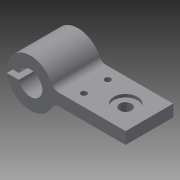
# Autodesk Inventor part: HW 5 Part 4
Saved by Autodesk Inventor 2015 (Build 190159000, 159)
## iProperties
Created: 2016-02-07
Part Number: HW 5 Part 4
Material: Generic
Document SubType Name: Modeling
Designer: Melissa
Density: 1 g/cm^3
Appearance: Default
Author: Melissa
Autodesk Inventor part; units mm, degrees
ref_plane "YZ Plane" through (0, 0, 0) normal (1, 0, 0) x (0, 1, 0)
ref_plane "XZ Plane" through (0, 0, 0) normal (0, 1, 0) x (-1, 0, 0)
ref_plane "XY Plane" through (0, 0, 0) normal (0, 0, 1) x (1, 0, 0)
sketch "Sketch1" plane through (0, 0, 0) normal (0, 0, 1) x (1, 0, 0)
  line L0 (4.5192, 0) -> (76.2, 0)
  line L1 (76.2, 0) -> (76.2, 12.7)
  line L2 (76.2, 12.7) -> (4.5192, 12.7)
  arc A0 (-37.6967, 3.175) -> (-37.6967, 9.525) centre (-25.4, 6.35) ccw
  arc A1 (-2.3852, 17.0962) -> (4.5192, 12.7) centre (4.5192, 20.32) ccw
  arc A2 (4.5192, 0) -> (-2.3852, -4.3962) centre (4.5192, -7.62) ccw
  line L3 (-50.6008, 9.525) -> (-38.1, 9.525)
  line L4 (-50.6008, 3.175) -> (-38.1, 3.175)
  line L5 (-38.1, 9.525) -> (-37.6967, 9.525)
  line L6 (-37.6967, 3.175) -> (-38.1, 3.175)
  arc A3 (-2.3852, 17.0962) -> (-50.6008, 9.525) centre (-25.4, 6.35) ccw
  arc A4 (-50.6008, 3.175) -> (-2.3852, -4.3962) centre (-25.4, 6.35) ccw
  point P0 (0, 0)
  dimension "d0" = 12.7
  dimension "d3" = 25.4
  dimension "d4" = 101.6
  dimension "d5" = 7.62
  dimension "d10" = 25.4
  constraints: 14 end point, 10 point on circle, 5 centre point, 2 horizontal, 2 tangent, 1 coincident, 1 equal radius, 1 parallel, 1 perpendicular, 1 point on line
  measures "d0" distance of L0.end L1.end
  measures "d3" diameter of A0
  measures "d4" horizontal distance of A3.centre L0.end
  measures "d5" radius of A1
  measures "d10" radius of A3
extrude "Extrusion1" add sketch "Sketch1" along normal blind 50.8
sketch "Sketch2" plane through (4.5192, 12.7, 0) normal (0, 1, 0) x (1, 0, 0)
  circle A0 centre (46.2808, -25.4) radius 6.35
  circle A1 centre (14.5308, -12.7) radius 3.175
  circle A2 centre (14.5308, -38.1) radius 3.175
  line L0 (71.6808, 0) -> (71.6808, -50.8) projected
  line L1 (0, 0) -> (71.6808, 0) projected
  line L2 (71.6808, -50.8) -> (0, -50.8) projected
  point P0 (-4.5192, 0)
  dimension "d13" = 12.7
  dimension "d14" = 6.35
  dimension "d15" = 6.35
  dimension "d16" = 25.4
  dimension "d17" = 25.4
  dimension "d18" = 57.15
  dimension "d19" = 12.7
  dimension "d20" = 25.4
  dimension "d21" = 0
  constraints: 3 centre point
  measures "d13" diameter of A0
  measures "d14" diameter of A1
  measures "d15" diameter of A2
  measures "d16" distance from line of L0 A0.centre
  measures "d17" distance from line of L1 A0.centre
  measures "d18" distance from line of L0 A2.centre
  measures "d19" distance from line of L2 A2.centre
  measures "d20" distance of A2.centre A1.centre
  measures "d21" horizontal distance of A2.centre A1.centre
extrude "Extrusion2" cut sketch "Sketch2" against normal through all
sketch "Sketch3" plane through (4.5192, 12.7, 0) normal (0, 1, 0) x (1, 0, 0)
  circle A0 centre (46.2808, -25.4) radius 6.35 projected
  circle A1 centre (46.2808, -25.4) radius 12.7
  point P0 (-4.5192, 0)
  dimension "d24" = 25.4
  constraints: 1 centre point, 1 coincident
  measures "d24" diameter of A1
extrude "Extrusion3" cut sketch "Sketch3" against normal blind 3.175
equation "\"d3\" = 2 * d0"
equation "\"d4\" = 8 * d0"
equation "\"d14\" = 0.5 * d13"
equation "\"d15\" = d14"
equation "\"d16\" = d17"
equation "\"d18\" = 2.25 * d16"
equation "\"d19\" = 0.5 * d17"
body "Solid1"
